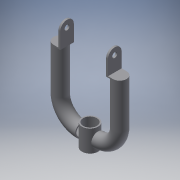
# Autodesk Inventor part: Wheel holder on handle bars axle
Saved by Autodesk Inventor 2018 (Build 220112000, 112)
## iProperties
Created: 2018-08-14
Part Number: Wheel holder on handle bars axle
Material: Generic
Document SubType Name: Modeling
Designer: ruben
Density: 1 g/cm^3
Sheet Metal Rule: Default_mm
Appearance: Default
Author: ruben
Autodesk Inventor part; units mm, degrees
ref_plane "YZ Plane" through (0, 0, 0) normal (1, 0, 0) x (0, 1, 0)
sketch "Sketch3" plane through (0, 0, 0) normal (0, 0, 1) x (1, 0, 0)
  line L0 (-18.2, 0) -> (18.2, 0) projected
  line L1 (0, -18.2) -> (0, 18.2) projected
  circle A0 centre (0, 0) radius 13
  circle A1 centre (0, 0) radius 11
  dimension "d0" = 26
  dimension "d1" = 22
  constraints: 2 centre point, 2 coincident
  measures "d0" diameter of A0
  measures "d1" diameter of A1
extrude "Extrusion1" add sketch "Sketch3" against normal blind 35 contours A1 L1 A0 L0 | L0 A0 L1 A1 | A1 L0 A0 L1 | L1 A0 L0 A1
ref_plane "Work Plane1" through (0, 13, 0) normal (0, 1, 0) x (-1, 0, 0)
sketch "Sketch4" plane through (0, 13, 0) normal (0, 1, 0) x (-1, 0, 0)
  line L0 (25.4907, 0) -> (-28.3112, 0) construction
  line L1 (21.6581, -35) -> (-31.1069, -35) construction
  line L2 (0, -47.4243) -> (0, 5.663) construction
  circle A0 centre (0, -17.5) radius 11
  circle A1 centre (0, -17.5) radius 9
  point P0 (0, 0)
  dimension "d4" = 35
  dimension "d5" = 17.5
  dimension "d9" = 22
  dimension "d10" = 18
  constraints: 6 end point, 3 point on line, 2 centre point, 2 coincident, 1 horizontal, 1 parallel, 1 perpendicular
  measures "d4" distance between parallel lines of L0 L1
  measures "d5" distance from line of L0 point (0, -17.5)
  measures "d9" diameter of A0
  measures "d10" diameter of A1
sketch3d "3D Sketch1"
  arc A0 (0, 13, -17.5) -> (0, 48, 17.5) centre (0, 13, 17.5) ccw
  line L0 (0, 48, 17.5) -> (0, 48, 87.5)
  dimension "d6" = 35
  dimension "d7" = 105
  dimension "d8" = 35
sweep "Sweep1" add profiles "Sketch4" path "3D Sketch1"
sketch "Sketch5" plane through (0, 48, 87.5) normal (0, 0, 1) x (1, 0, 0)
  line L0 (11, 0) -> (11, -11)
  line L1 (11, -11) -> (-11, -11)
  line L2 (-11, -11) -> (-11, 0)
  line L3 (-11, 11) -> (11, -11) construction
  line L4 (11, 11) -> (-11, -11) construction
  arc A0 (11, 0) -> (-11, 0) centre (0, 0) ccw
  point P0 (0, -48)
  dimension "d13" = 22
  dimension "d14" = 22
  constraints: 10 end point, 2 midpoint, 2 point on circle, 1 centre point, 1 coincident, 1 parallel
  measures "d13" distance of L0.end L1.end
  measures "d14" distance of L4.start L0.end
extrude "Extrusion2" add sketch "Sketch5" along normal blind 2
sketch "Sketch6" plane through (0, 48, 89.5) normal (0, 0, 1) x (1, 0, 0)
  line L0 (0, -11) -> (11, -11) projected
  line L1 (-11, 0) -> (-11, -11) projected
  line L2 (11, -11) -> (-11, -11)
  line L3 (-11, -11) -> (-11, -8)
  line L4 (-11, -8) -> (11, -8)
  line L5 (11, -8) -> (11, -11)
  point P0 (0, -48)
  dimension "d17" = 3
  constraints: 8 end point, 2 parallel, 1 horizontal, 1 perpendicular, 1 point on line
  measures "d17" distance of L2.end L3.end
extrude "Extrusion3" add sketch "Sketch6" along normal blind 35
sketch "Sketch7" plane through (-11, 37, 87.5) normal (0, -1, 0) x (1, 0, 0)
  line L0 (22, 0) -> (22, 37) projected
  line L1 (0, 0) -> (0, 37) projected
  arc A0 (22, 26) -> (0, 26) centre (11, 26) ccw
  line L2 (0, 37) -> (22, 37) projected
  point P0 (11, -87.5)
  point P1 (11, 37)
  dimension "d20" = 11
  constraints: 3 point on circle, 2 point on line, 1 centre point, 1 midpoint
  measures "d20" radius of A0
extrude "Extrusion4" cut sketch "Sketch7" against normal up to surface (3 mm away)
sketch "Sketch8" plane through (-11, 40, 89.5) normal (0, 1, 0) x (1, 0, 0)
  circle A0 centre (11, -24) radius 4
  arc A1 (0, -24) -> (22, -24) centre (11, -24) ccw projected
  point P0 (11, 89.5)
  dimension "d23" = 8
  dimension "d24" = 0
  constraints: 1 centre point, 1 coincident
  measures "d23" diameter of A0
  measures "d24" distance of A1.centre A0.centre
extrude "Extrusion5" cut sketch "Sketch8" against normal up to next
ref_plane "Work Plane2" through (0, -13, 0) normal (0, 1, 0) x (-1, 0, 0)
sketch "Sketch11" plane through (0, -13, 0) normal (0, 1, 0) x (-1, 0, 0)
  line L0 (25.4907, 0) -> (-28.3112, 0) construction
  line L1 (21.6581, -35) -> (-31.1069, -35) construction
  line L2 (0, -47.4243) -> (0, 5.663) construction
  circle A0 centre (0, -17.5) radius 11
  circle A1 centre (0, -17.5) radius 9
  point P0 (0, 0)
  dimension "d27" = 35
  dimension "d28" = 17.5
  dimension "d29" = 22
  dimension "d30" = 18
  constraints: 6 end point, 3 point on line, 2 centre point, 2 coincident, 1 horizontal, 1 parallel, 1 perpendicular
  measures "d27" distance between parallel lines of L0 L1
  measures "d28" distance from line of L0 point (0, -17.5)
  measures "d29" diameter of A0
  measures "d30" diameter of A1
sketch3d "3D Sketch2"
  arc A0 (0, -13, -17.5) -> (0, -48, 17.5) centre (0, -13, 17.5) ccw
  line L0 (0, -48, 17.5) -> (0, -48, 87.5)
  dimension "d31" = 35
  dimension "d32" = 105
  dimension "d33" = 35
sweep "Sweep2" add profiles "Sketch11" path "3D Sketch2"
sketch "Sketch12" plane through (0, -48, 87.5) normal (0, 0, 1) x (1, 0, 0)
  line L0 (-11, 11) -> (11, 11)
  line L1 (11, 11) -> (11, 0)
  line L2 (-11, 0) -> (-11, 11)
  line L3 (-11, 11) -> (11, -11) construction
  line L4 (11, 11) -> (-11, -11) construction
  arc A0 (-11, 0) -> (11, 0) centre (0, 0) ccw
  point P0 (0, 48)
  dimension "d40" = 22
  dimension "d41" = 22
  constraints: 10 end point, 2 midpoint, 2 point on circle, 1 centre point, 1 coincident, 1 horizontal, 1 parallel, 1 perpendicular
  measures "d40" distance of L3.end L0.end
  measures "d41" distance of L4.end L3.end
extrude "Extrusion6" add sketch "Sketch12" along normal blind 2
sketch "Sketch13" plane through (0, -48, 89.5) normal (0, 0, 1) x (1, 0, 0)
  line L0 (0, 11) -> (11, 11) projected
  line L1 (11, 11) -> (-11, 11)
  line L2 (-11, 11) -> (-11, 8)
  line L3 (-11, 8) -> (11, 8)
  line L4 (11, 8) -> (11, 11)
  point P0 (0, 48)
  dimension "d44" = 22
  dimension "d45" = 3
  constraints: 8 end point, 2 parallel, 1 horizontal, 1 perpendicular
  measures "d44" distance of L3.end L2.end
  measures "d45" distance of L2.end L1.end
extrude "Extrusion7" add sketch "Sketch13" along normal blind 35
extrude "Extrusion8" cut sketch "Sketch7" along normal up to surface (77 mm away)
sketch "Sketch16" plane through (-11, -40, 89.5) normal (0, -1, 0) x (1, 0, 0)
  circle A0 centre (11, 24) radius 4 projected
  circle A1 centre (11, 24) radius 4
  point P0 (11, -89.5)
  dimension "d53" = 8
  constraints: 2 coincident, 1 centre point
  measures "d53" diameter of A1
extrude "Extrusion9" cut sketch "Sketch16" against normal up to next
equation "\"d5\" = 0.5 * d4"
equation "\"d13\" = d14"
equation "\"d28\" = 0.5 * d27"
equation "\"d41\" = d40"
equation "\"BendRadius\" = Thickness"
equation "\"BendReliefWidth\" = Thickness"
equation "\"BendReliefDepth\" = 0.5 * Thickness"
equation "\"CornerReliefSize\" = 4 * Thickness"
equation "\"MinimumRemnant\" = 2 * Thickness"
equation "\"TransitionRadius\" = BendRadius"
equation "\"JacobiRadiusSize\" = BendRadius"
equation "\"GapSize\" = Thickness"
equation "\"Thickness\" = 0.5"
body "Solid1"
